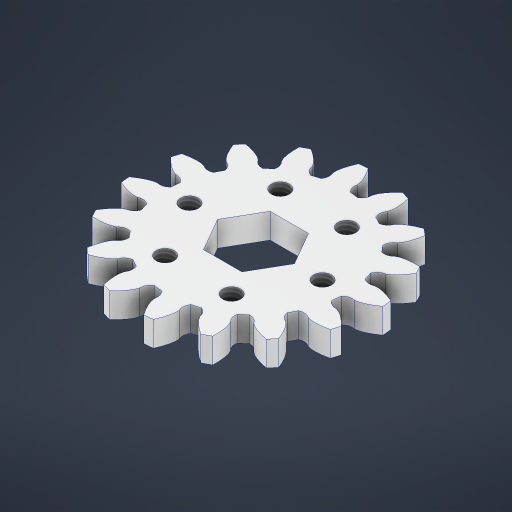
# Autodesk Inventor part: CLIM_006_RackGear
Saved by Autodesk Inventor 2024.2 (Build 282272000, 272)
## iProperties
Created: 2024-08-08
Part Number: CLIM_006_RackGear
Material: Aluminum 6061
Document SubType Name: Modeling
Designer: Bryan
Density: 2.7 g/cm^3
Appearance: Aluminum - Flat
Author: Bryan
Autodesk Inventor part; units mm, degrees
ref_plane "YZ Plane" through (0, 0, 0) normal (1, 0, 0) x (0, 1, 0)
ref_plane "XZ Plane" through (0, 0, 0) normal (0, 1, 0) x (-1, 0, 0)
ref_plane "XY Plane" through (0, 0, 0) normal (0, 0, 1) x (1, 0, 0)
sketch "Sketch1" plane through (0, 0, 0) normal (0, 1, 0) x (-1, 0, 0)
  circle A0 centre (0, 0) radius 20.32 construction
  circle A1 centre (0, 0) radius 17.145
  circle A2 centre (0, 0) radius 22.86
  line L0 (0, 0) -> (20.32, 0) construction
  line L1 (20.32, 0) -> (17.943, 6.5307) construction
  line L2 (17.943, 6.5307) -> (0, 0) construction
  arc A3 (19.0924, -0.2846) -> (17.943, 6.5307) centre (0, 0) ccw construction
  arc A4 (17.943, 6.5307) -> (15.2775, 11.4543) centre (0, 0) ccw construction
  line L3 (15.2775, 11.4543) -> (22.8172, 1.398) construction
  line L4 (17.9053, 14.212) -> (16.3387, -15.9883) construction
  line L5 (19.0924, -0.2846) -> (17.122, -0.8882) construction
  line L6 (21.1231, 8.7404) -> (11.3123, -19.8649) construction
  line L7 (19.0924, -0.2846) -> (18.0209, -0.3046) construction
  line L8 (18.0209, -0.3046) -> (17.122, -0.8882) construction
  spline S0 degree 2 poles (22.8172, 1.398) (20.4165, -0.2494) (19.0924, -0.2846) knots 0 0 0 1 1 1
  spline S1 degree 2 poles (19.0924, -0.2846) (17.9346, -0.0228) (17.122, -0.8882) knots 0 0 0 1 1 1
  line L9 (0, 0) -> (17.0624, -1.6805) construction
  spline S2 degree 2 poles (22.1061, -5.8225) (20.0728, -3.7385) (18.7811, -3.4456) knots 0 0 0 1 1 1
  spline S3 degree 2 poles (18.7811, -3.4456) (17.5944, -3.4765) (16.9663, -2.4692) knots 0 0 0 1 1 1
  spline S4 degree 2 poles (20.5454, 10.0233) (18.9578, 7.5826) (17.748, 7.0434) knots 0 0 0 1 1 1
  spline S5 degree 2 poles (17.748, 7.0434) (16.5781, 6.8422) (16.1585, 5.7317) knots 0 0 0 1 1 1
  spline S6 degree 2 poles (18.6701, 4.0039) (17.5855, 3.5212) (16.6197, 4.2114) knots 0 0 0 1 1 1
  spline S7 degree 2 poles (22.6515, 3.0803) (19.9755, 4.2276) (18.6701, 4.0039) knots 0 0 0 1 1 1
  spline S8 degree 2 poles (15.1457, 17.1227) (14.613, 14.2603) (13.7016, 13.2992) knots 0 0 0 1 1 1
  spline S9 degree 2 poles (13.7016, 13.2992) (12.6978, 12.6655) (12.7351, 11.479) knots 0 0 0 1 1 1
  spline S10 degree 2 poles (15.7167, 10.8438) (14.8994, 9.9829) (13.743, 10.2509) knots 0 0 0 1 1 1
  spline S11 degree 2 poles (19.7485, 11.5142) (16.8371, 11.5501) (15.7167, 10.8438) knots 0 0 0 1 1 1
  spline S12 degree 2 poles (7.4402, 21.6153) (8.0434, 18.7669) (7.5693, 17.5302) knots 0 0 0 1 1 1
  spline S13 degree 2 poles (7.5693, 17.5302) (6.8843, 16.5607) (7.3729, 15.4788) knots 0 0 0 1 1 1
  spline S14 degree 2 poles (10.3706, 16.0329) (9.945, 14.9247) (8.774, 14.7298) knots 0 0 0 1 1 1
  spline S15 degree 2 poles (13.8389, 18.1952) (11.1354, 17.1142) (10.3706, 16.0329) knots 0 0 0 1 1 1
  spline S16 degree 2 poles (-1.398, 22.8172) (0.2494, 20.4165) (0.2846, 19.0924) knots 0 0 0 1 1 1
  spline S17 degree 2 poles (0.2846, 19.0924) (0.0228, 17.9346) (0.8882, 17.122) knots 0 0 0 1 1 1
  spline S18 degree 2 poles (3.4456, 18.7811) (3.4765, 17.5944) (2.4692, 16.9663) knots 0 0 0 1 1 1
  spline S19 degree 2 poles (5.8225, 22.1061) (3.7385, 20.0728) (3.4456, 18.7811) knots 0 0 0 1 1 1
  spline S20 degree 2 poles (-10.0233, 20.5454) (-7.5826, 18.9578) (-7.0434, 17.748) knots 0 0 0 1 1 1
  spline S21 degree 2 poles (-7.0434, 17.748) (-6.8422, 16.5781) (-5.7317, 16.1585) knots 0 0 0 1 1 1
  spline S22 degree 2 poles (-4.0039, 18.6701) (-3.5212, 17.5855) (-4.2114, 16.6197) knots 0 0 0 1 1 1
  spline S23 degree 2 poles (-3.0803, 22.6515) (-4.2276, 19.9755) (-4.0039, 18.6701) knots 0 0 0 1 1 1
  spline S24 degree 2 poles (-17.1227, 15.1457) (-14.2603, 14.613) (-13.2992, 13.7016) knots 0 0 0 1 1 1
  spline S25 degree 2 poles (-13.2992, 13.7016) (-12.6655, 12.6978) (-11.479, 12.7351) knots 0 0 0 1 1 1
  spline S26 degree 2 poles (-10.8438, 15.7167) (-9.9829, 14.8994) (-10.2509, 13.743) knots 0 0 0 1 1 1
  spline S27 degree 2 poles (-11.5142, 19.7485) (-11.5501, 16.8371) (-10.8438, 15.7167) knots 0 0 0 1 1 1
  spline S28 degree 2 poles (-21.6153, 7.4402) (-18.7669, 8.0434) (-17.5302, 7.5693) knots 0 0 0 1 1 1
  spline S29 degree 2 poles (-17.5302, 7.5693) (-16.5607, 6.8843) (-15.4788, 7.3729) knots 0 0 0 1 1 1
  spline S30 degree 2 poles (-16.0329, 10.3706) (-14.9247, 9.945) (-14.7298, 8.774) knots 0 0 0 1 1 1
  spline S31 degree 2 poles (-18.1952, 13.8389) (-17.1142, 11.1354) (-16.0329, 10.3706) knots 0 0 0 1 1 1
  spline S32 degree 2 poles (-22.8172, -1.398) (-20.4165, 0.2494) (-19.0924, 0.2846) knots 0 0 0 1 1 1
  spline S33 degree 2 poles (-19.0924, 0.2846) (-17.9346, 0.0228) (-17.122, 0.8882) knots 0 0 0 1 1 1
  spline S34 degree 2 poles (-18.7811, 3.4456) (-17.5944, 3.4765) (-16.9663, 2.4692) knots 0 0 0 1 1 1
  spline S35 degree 2 poles (-22.1061, 5.8225) (-20.0728, 3.7385) (-18.7811, 3.4456) knots 0 0 0 1 1 1
  spline S36 degree 2 poles (-20.5454, -10.0233) (-18.9578, -7.5826) (-17.748, -7.0434) knots 0 0 0 1 1 1
  spline S37 degree 2 poles (-17.748, -7.0434) (-16.5781, -6.8422) (-16.1585, -5.7317) knots 0 0 0 1 1 1
  spline S38 degree 2 poles (-18.6701, -4.0039) (-17.5855, -3.5212) (-16.6197, -4.2114) knots 0 0 0 1 1 1
  spline S39 degree 2 poles (-22.6515, -3.0803) (-19.9755, -4.2276) (-18.6701, -4.0039) knots 0 0 0 1 1 1
  spline S40 degree 2 poles (-15.1457, -17.1227) (-14.613, -14.2603) (-13.7016, -13.2992) knots 0 0 0 1 1 1
  spline S41 degree 2 poles (-13.7016, -13.2992) (-12.6978, -12.6655) (-12.7351, -11.479) knots 0 0 0 1 1 1
  spline S42 degree 2 poles (-15.7167, -10.8438) (-14.8994, -9.9829) (-13.743, -10.2509) knots 0 0 0 1 1 1
  spline S43 degree 2 poles (-19.7485, -11.5142) (-16.8371, -11.5501) (-15.7167, -10.8438) knots 0 0 0 1 1 1
  spline S44 degree 2 poles (-7.4402, -21.6153) (-8.0434, -18.7669) (-7.5693, -17.5302) knots 0 0 0 1 1 1
  spline S45 degree 2 poles (-7.5693, -17.5302) (-6.8843, -16.5607) (-7.3729, -15.4788) knots 0 0 0 1 1 1
  spline S46 degree 2 poles (-10.3706, -16.0329) (-9.945, -14.9247) (-8.774, -14.7298) knots 0 0 0 1 1 1
  spline S47 degree 2 poles (-13.8389, -18.1952) (-11.1354, -17.1142) (-10.3706, -16.0329) knots 0 0 0 1 1 1
  spline S48 degree 2 poles (1.398, -22.8172) (-0.2494, -20.4165) (-0.2846, -19.0924) knots 0 0 0 1 1 1
  spline S49 degree 2 poles (-0.2846, -19.0924) (-0.0228, -17.9346) (-0.8882, -17.122) knots 0 0 0 1 1 1
  spline S50 degree 2 poles (-3.4456, -18.7811) (-3.4765, -17.5944) (-2.4692, -16.9663) knots 0 0 0 1 1 1
  spline S51 degree 2 poles (-5.8225, -22.1061) (-3.7385, -20.0728) (-3.4456, -18.7811) knots 0 0 0 1 1 1
  spline S52 degree 2 poles (10.0233, -20.5454) (7.5826, -18.9578) (7.0434, -17.748) knots 0 0 0 1 1 1
  spline S53 degree 2 poles (7.0434, -17.748) (6.8422, -16.5781) (5.7317, -16.1585) knots 0 0 0 1 1 1
  spline S54 degree 2 poles (4.0039, -18.6701) (3.5212, -17.5855) (4.2114, -16.6197) knots 0 0 0 1 1 1
  spline S55 degree 2 poles (3.0803, -22.6515) (4.2276, -19.9755) (4.0039, -18.6701) knots 0 0 0 1 1 1
  spline S56 degree 2 poles (17.1227, -15.1457) (14.2603, -14.613) (13.2992, -13.7016) knots 0 0 0 1 1 1
  spline S57 degree 2 poles (13.2992, -13.7016) (12.6655, -12.6978) (11.479, -12.7351) knots 0 0 0 1 1 1
  spline S58 degree 2 poles (10.8438, -15.7167) (9.9829, -14.8994) (10.2509, -13.743) knots 0 0 0 1 1 1
  spline S59 degree 2 poles (11.5142, -19.7485) (11.5501, -16.8371) (10.8438, -15.7167) knots 0 0 0 1 1 1
  spline S60 degree 2 poles (21.6153, -7.4402) (18.7669, -8.0434) (17.5302, -7.5693) knots 0 0 0 1 1 1
  spline S61 degree 2 poles (17.5302, -7.5693) (16.5607, -6.8843) (15.4788, -7.3729) knots 0 0 0 1 1 1
  spline S62 degree 2 poles (16.0329, -10.3706) (14.9247, -9.945) (14.7298, -8.774) knots 0 0 0 1 1 1
  spline S63 degree 2 poles (18.1952, -13.8389) (17.1142, -11.1354) (16.0329, -10.3706) knots 0 0 0 1 1 1
  line L10 (-3.6662, 6.35) -> (3.6662, 6.35)
  line L11 (3.6662, 6.35) -> (7.3323, 0)
  line L12 (7.3323, 0) -> (3.6662, -6.35)
  line L13 (3.6662, -6.35) -> (-3.6662, -6.35)
  line L14 (-3.6662, -6.35) -> (-7.3323, 0)
  line L15 (-7.3323, 0) -> (-3.6662, 6.35)
  point P0 (19.9296, -3.9642)
  point P1 (17.734, -3.217)
  point P2 (18.7732, 7.7761)
  point P3 (16.7657, 6.6149)
  point P4 (17.6152, 3.8144)
  point P5 (19.9296, 3.9642)
  point P6 (14.3684, 14.3684)
  point P7 (12.9581, 12.5273)
  point P8 (14.8146, 10.2651)
  point P9 (16.8955, 11.2892)
  point P10 (7.7761, 18.7732)
  point P11 (7.1777, 16.5326)
  point P12 (9.7586, 15.153)
  point P13 (11.2892, 16.8955)
  point P14 (0, 20.32)
  point P15 (0.3046, 18.0209)
  point P16 (3.217, 17.734)
  point P17 (3.9642, 19.9296)
  point P18 (-7.7761, 18.7732)
  point P19 (-6.6149, 16.7657)
  point P20 (-3.8144, 17.6152)
  point P21 (-3.9642, 19.9296)
  point P22 (-14.3684, 14.3684)
  point P23 (-12.5273, 12.9581)
  point P24 (-10.2651, 14.8146)
  point P25 (-11.2892, 16.8955)
  point P26 (-18.7732, 7.7761)
  point P27 (-16.5326, 7.1777)
  point P28 (-15.153, 9.7586)
  point P29 (-16.8955, 11.2892)
  point P30 (-20.32, 0)
  point P31 (-18.0209, 0.3046)
  point P32 (-17.734, 3.217)
  point P33 (-19.9296, 3.9642)
  point P34 (-18.7732, -7.7761)
  point P35 (-16.7657, -6.6149)
  point P36 (-17.6152, -3.8144)
  point P37 (-19.9296, -3.9642)
  point P38 (-14.3684, -14.3684)
  point P39 (-12.9581, -12.5273)
  point P40 (-14.8146, -10.2651)
  point P41 (-16.8955, -11.2892)
  point P42 (-7.7761, -18.7732)
  point P43 (-7.1777, -16.5326)
  point P44 (-9.7586, -15.153)
  point P45 (-11.2892, -16.8955)
  point P46 (0, -20.32)
  point P47 (-0.3046, -18.0209)
  point P48 (-3.217, -17.734)
  point P49 (-3.9642, -19.9296)
  point P50 (7.7761, -18.7732)
  point P51 (6.6149, -16.7657)
  point P52 (3.8144, -17.6152)
  point P53 (3.9642, -19.9296)
  point P54 (14.3684, -14.3684)
  point P55 (12.5273, -12.9581)
  point P56 (10.2651, -14.8146)
  point P57 (11.2892, -16.8955)
  point P58 (18.7732, -7.7761)
  point P59 (16.5326, -7.1777)
  point P60 (15.153, -9.7586)
  point P61 (16.8955, -11.2892)
  point P62 (16.1585, 5.7317)
  point P63 (12.7351, 11.479)
  point P64 (7.3729, 15.4788)
  point P65 (0.8882, 17.122)
  point P66 (-1.398, 22.8172)
  point P67 (-4.2114, 16.6197)
  point P68 (-5.7317, 16.1585)
  point P69 (-11.479, 12.7351)
  point P70 (-15.4788, 7.3729)
  point P71 (-16.9663, 2.4692)
  point P72 (-17.122, 0.8882)
  point P73 (-22.8172, -1.398)
  point P74 (-16.1585, -5.7317)
  point P75 (-12.7351, -11.479)
  point P76 (-7.3729, -15.4788)
  point P77 (-2.4692, -16.9663)
  point P78 (-0.8882, -17.122)
  point P79 (1.398, -22.8172)
  point P80 (4.2114, -16.6197)
  point P81 (5.7317, -16.1585)
  point P82 (11.479, -12.7351)
  point P83 (15.4788, -7.3729)
  point P84 (16.9663, -2.4692)
  point P85 (17.122, -0.8882)
  dimension "d0" = 40.64
  dimension "d1" = 34.29
  dimension "d2" = 45.72
  dimension "d3" = 20
  dimension "d4" = 6.9498
  dimension "d5" = 6.9498
  dimension "d6" = 12.5689
  dimension "d7" = 5.6191
  dimension "d8" = 70
  dimension "d9" = 70
  dimension "d10" = 5.625
  dimension "d13" = 360
  dimension "d15" = 12.7
  constraints: 32 end point, 5 symmetric about line, 4 coincident, 4 point on circle, 2 centre point, 2 horizontal, 1 equal length, 1 horizontal alignment, 1 midpoint, 1 perpendicular, 1 point on line, 1 tangent, 446 other
  measures "d3" angle of L0 L2
  measures "d4" distance of L0.end L1.end
  measures "d6" distance of L3.start L3.end
  measures "d8" angle of L4 L5
  measures "d9" angle of L6 L7
  measures "d10" angle of L9 L0
  measures "d15" distance between parallel lines of L13 L10
extrude "Extrusion1" add sketch "Sketch1" along normal blind 4.7625 contours A1 | A1 S6 S7 A2 S0 S1 | A1 S10 S11 A2 S4 S5 | S3 S2 A2 S60 S61 A1 | A1 S14 S15 A2 S8 S9 | S62 S63 A2 S56 S57 A1 | A1 S18 S19 A2 S12 S13 | S58 S59 A2 S52 S53 A1 | A1 S22 S23 A2 S16 S17 | S54 S55 A2 S48 S49 A1 | A1 S26 S27 A2 S20 S21 | S50 S51 A2 S44 S45 A1 | A1 S30 S31 A2 S24 S25 | S46 S47 A2 S40 S41 A1 | A1 S34 S35 A2 S28 S29 | S42 S43 A2 S36 S37 A1 | A1 S38 S39 A2 S32 S33
sketch "Sketch2" plane through (0, 4.7625, 0) normal (0, 1, 0) x (1, 0, 0)
  line L0 (0, 0) -> (-12.7, 0)
  circle A0 centre (-12.7, 0) radius 1.7145
  circle A1 centre (-6.35, -10.9985) radius 1.7145
  circle A2 centre (6.35, -10.9985) radius 1.7145
  circle A3 centre (12.7, 0) radius 1.7145
  circle A4 centre (6.35, 10.9985) radius 1.7145
  circle A5 centre (-6.35, 10.9985) radius 1.7145
  dimension "d18" = 12.7
  dimension "d19" = 3.429
  dimension "d22" = 360
  constraints: 6 centre point, 2 end point, 1 coincident, 1 horizontal, 13 other
  measures "d18" distance of L0.start L0.end
  measures "d19" diameter of A0
extrude "Extrusion2" cut sketch "Sketch2" against normal blind 4.7625
thread "Thread1" size "8-32 UNC" class "2B" standard "ANSI Unified Screw Threads" full length
thread "Thread2" size "8-32 UNC" class "2B" standard "ANSI Unified Screw Threads" full length
thread "Thread3" size "8-32 UNC" class "2B" standard "ANSI Unified Screw Threads" full length
thread "Thread4" size "8-32 UNC" class "2B" standard "ANSI Unified Screw Threads" full length
thread "Thread5" size "8-32 UNC" class "2B" standard "ANSI Unified Screw Threads" full length
thread "Thread6" size "8-32 UNC" class "2B" standard "ANSI Unified Screw Threads" full length
equation "\"d0\" = pd"
equation "\"d1\" = rd"
equation "\"d2\" = od"
equation "\"d3\" = a"
equation "\"d5\" = d4"
equation "\"d7\" = d6 - d4"
equation "\"a\" = 20deg"
equation "\"ded\" = 1.25 * mod"
equation "\"od\" = pd + 2 * mod"
equation "\"rd\" = pd - 2 * ded"
equation "\"pd\" = 40.64"
equation "\"mod\" = 2.54"
body "Solid1"
